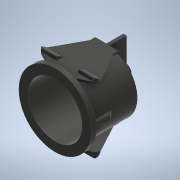
# Autodesk Inventor part: body
Saved by Autodesk Inventor 2022.1 (Build 261234000, 234)
## iProperties
Created: 2019-08-22
Part Number: body
Material: Пластмасса, непрозрачная, черная
Document SubType Name: Modeling
Designer: Иванов Д.А.
Mass: 3.57903 g
Surface Area: 53.3584 cm^2
Volume: 3.75948 cm^3
Density: 0.952 g/cm^3
Appearance: Гладкая — черная
Author: Иванов Д.А.
Autodesk Inventor part; units mm, degrees
ref_plane "YZ Plane" through (0, 0, 0) normal (1, 0, 0) x (0, 1, 0)
ref_plane "XZ Plane" through (0, 0, 0) normal (0, 1, 0) x (-1, 0, 0)
sketch "Эскиз1" plane through (0, 0, 0) normal (0, 1, 0) x (-1, 0, 0)
  circle A0 centre (0, 0) radius 11.75
  dimension "d0" = 23.5
  constraints: 1 centre point, 1 coincident
  measures "d0" diameter of A0
extrude "Выдавливание1" add sketch "Эскиз1" along normal blind 18
sketch "Эскиз2" plane through (0, 0, 0) normal (0, -1, 0) x (1, 0, 0)
  circle A0 centre (0, 0) radius 14
  dimension "d3" = 28
  constraints: 1 centre point, 1 coincident
  measures "d3" diameter of A0
extrude "Выдавливание2" add sketch "Эскиз2" along normal blind 2
sketch "Эскиз3" plane through (0, 18, 0) normal (0, 1, 0) x (1, 0, 0)
  line L0 (0, 11.75) -> (0, -11.75) construction
  line L1 (-0.6, 11.7347) -> (-0.6, 2.4269)
  line L2 (0.6, 11.7347) -> (0.6, 2.4269)
  line L3 (-11.75, 0) -> (11.75, 0) construction
  line L4 (-0.6, -11.7347) -> (-0.6, -2.4269)
  line L5 (0.6, -11.7347) -> (0.6, -2.4269)
  arc A0 (-0.6, 2.4269) -> (-0.6, -2.4269) centre (0, 0) ccw
  arc A1 (0.6, -2.4269) -> (0.6, 2.4269) centre (0, 0) ccw
  circle A2 centre (0, 0) radius 11.75 projected
  line L6 (-11.3865, 2.9) -> (-4.75, 2.9)
  line L7 (-4.75, 2.9) -> (-4.75, -2.9)
  line L8 (-4.75, -2.9) -> (-11.3865, -2.9)
  line L9 (-7.75, 1.9) -> (-5.75, 1.9)
  line L10 (-5.75, 1.9) -> (-5.75, -1.9)
  line L11 (-5.75, -1.9) -> (-7.75, -1.9)
  line L12 (-7.75, -1.9) -> (-7.75, 1.9)
  dimension "d7" = 1.2
  dimension "d8" = 2.5
  dimension "d12" = 5.8
  dimension "d13" = 7
  dimension "d14" = 1
  dimension "d15" = 1
  dimension "d16" = 1
  dimension "d17" = 2
  constraints: 26 end point, 4 point on circle, 3 midpoint, 3 symmetric about line, 2 centre point, 2 collinear, 2 perpendicular, 1 coincident, 1 vertical, 12 other
  measures "d7" diameter of L1 L0
  measures "d8" radius of A1
  measures "d12" distance between parallel lines of L8 L6
  measures "d13" distance from line of L3.start L7
  measures "d14" distance between parallel lines of L7 L10
  measures "d15" distance between parallel lines of L6 L9
  measures "d16" distance between parallel lines of L8 L11
  measures "d17" distance between parallel lines of L12 L10
extrude "Выдавливание3" add sketch "Эскиз3" along normal blind 7 contours A2 L2 A1 L5 L4 A0 L1 | L6 L7 L8 A2
sketch "Эскиз4" plane through (0, -2, 0) normal (0, -1, 0) x (1, 0, 0)
  circle A0 centre (0, 0) radius 10.5
  dimension "d18" = 21
  constraints: 1 centre point, 1 coincident
  measures "d18" diameter of A0
extrude "Выдавливание4" cut sketch "Эскиз4" against normal blind 18
sketch "Эскиз5" plane through (0, 0, 0) normal (0, 1, 0) x (1, 0, 0)
  arc A0 (0.6, -11.7347) -> (0.6, 11.7347) centre (0, 0) ccw projected
  line L0 (11.7155, 0.9) -> (12.95, 0.9)
  line L1 (12.95, 0.9) -> (12.95, -0.9)
  line L2 (12.95, -0.9) -> (11.7155, -0.9)
  line L3 (0, 0) -> (19.973, 0) construction
  point P0 (11.75, 0)
  point P1 (11.75, 0)
  dimension "d21" = 1.8
  dimension "d22" = 1.2
  constraints: 8 end point, 4 point on circle, 2 point on line, 1 horizontal, 1 perpendicular, 1 other
  measures "d21" distance between parallel lines of L2 L0
  measures "d22" distance from line of L1 point (11.75, 0)
extrude "Выдавливание5" add sketch "Эскиз5" along normal blind 8
chamfer "Фаска1" distance 1.7 angle 35 1 edges at (12.95, 8, 0) measured on face at (12.95, 2.6667, -0.3)
ref_plane "РабПлоскость1" through (0, 0, 11.75) normal (0, 0, 1) x (1, 0, 0)
sketch "Эскиз7" plane through (0, 0, 11.75) normal (0, 0, 1) x (1, 0, 0)
  line L0 (11.75, 18) -> (0.6, 18) projected
  line L1 (-0.6, 18) -> (-11.3865, 18) projected
  line L2 (0, 18) -> (4.5, 18)
  line L3 (4.5, 18) -> (4.5, 16)
  line L4 (4.5, 0) -> (0, 0)
  line L5 (14, 0) -> (-14, 0) projected
  line L6 (0.6, 18) -> (-0.6, 18) construction
  line L7 (0, 18) -> (0, 0) construction
  line L8 (4.5, 0) -> (9.9502, 2.6511)
  line L9 (10.613, 4.7144) -> (4.5, 16)
  arc A0 (9.9502, 2.6511) -> (10.613, 4.7144) centre (9.2941, 4) ccw
  line L10 (0, 18) -> (-4.5, 18)
  line L11 (-4.5, 18) -> (-4.5, 16)
  line L12 (-4.5, 0) -> (0, 0)
  line L13 (-4.5, 0) -> (-9.9502, 2.6511)
  line L14 (-10.613, 4.7144) -> (-4.5, 16)
  arc A1 (-10.613, 4.7144) -> (-9.9502, 2.6511) centre (-9.2941, 4) ccw
  point P0 (11, 4)
  dimension "d30" = 9
  dimension "d31" = 4
  dimension "d32" = 22
  dimension "d33" = 1.5
  dimension "d34" = 2
  dimension "d35" = 154.061
  constraints: 24 end point, 6 symmetric about line, 4 point on circle, 2 centre point, 2 collinear, 2 midpoint, 2 tangent, 1 horizontal alignment, 1 point on line, 1 other
  measures "d30" diameter of L3 L7
  measures "d31" distance from line of L5 point (11, 4)
  measures "d32" diameter of point (11, 4) L7
  measures "d33" radius of A0
  measures "d34" distance from line of L3.end L0
  measures "d35" angle of L4 L8
extrude "Выдавливание6" add sketch "Эскиз7" along normal mid plane 0.8
mirror "Зеркальное отражение1" about plane through (0, 0, 0) normal (0, 0, 1) of "Выдавливание6"
sketch "Эскиз9" plane through (0, 0, 12.15) normal (0, 0, 1) x (1, 0, 0)
  line L0 (4.5, 0) -> (-4.5, 0) projected
  line L1 (4.5, 0) -> (9.9502, 2.6511) projected
  arc A0 (9.9502, 2.6511) -> (10.613, 4.7144) centre (9.2941, 4) ccw projected
  line L2 (10.613, 4.7144) -> (4.5, 16) projected
  line L3 (4.5, 16) -> (4.5, 18) projected
  line L4 (4.5, 18) -> (-4.5, 18) projected
  line L5 (-4.5, 18) -> (-4.5, 16) projected
  line L6 (-4.5, 16) -> (-10.613, 4.7144) projected
  arc A1 (-10.613, 4.7144) -> (-9.9502, 2.6511) centre (-9.2941, 4) ccw projected
  line L7 (-9.9502, 2.6511) -> (-4.5, 0) projected
  line L8 (4.2, 5.25) -> (10.3229, 5.25)
  line L9 (10.1232, 2.75) -> (4.2, 2.75)
  line L10 (4.2, 2.75) -> (4.2, 5.25)
  line L11 (0, 18) -> (0, 0) construction
  line L12 (9.2941, 4) -> (-9.2941, 4) construction
  arc A2 (-10.613, 4.7144) -> (-9.9502, 2.6511) centre (-9.2941, 4) ccw
  line L13 (-4.2, 5.25) -> (-10.3229, 5.25)
  line L14 (-10.1232, 2.75) -> (-4.2, 2.75)
  line L15 (-4.2, 2.75) -> (-4.2, 5.25)
  dimension "d40" = 4.2
  dimension "d43" = 2.5
  constraints: 16 end point, 4 point on circle, 2 collinear, 2 point on line, 2 symmetric about line, 1 centre point, 1 midpoint, 2 other
  measures "d40" distance between parallel lines of L11 L10
  measures "d43" distance between parallel lines of L9 L8
extrude "Выдавливание8" add sketch "Эскиз9" along normal blind 1.2 contours L9 L10 L8 L2 A0 | A1 L6 L13 L15 L14
chamfer "Фаска2" distance 2.05 angle 30 1 edges at (7.2615, 5.25, 13.35) measured on face at (8.2154, 4.4167, 13.35)
chamfer "Фаска3" distance 2.05 angle 30 1 edges at (-7.2615, 5.25, 13.35) measured on face at (-8.2154, 4.4167, 13.35)
mirror "Зеркальное отражение2" about plane through (0, 0, 0) normal (0, 0, 1) of "Выдавливание8", "Фаска2", "Фаска3"
equation "\"d15\" = d14"
equation "\"d16\" = d14"
